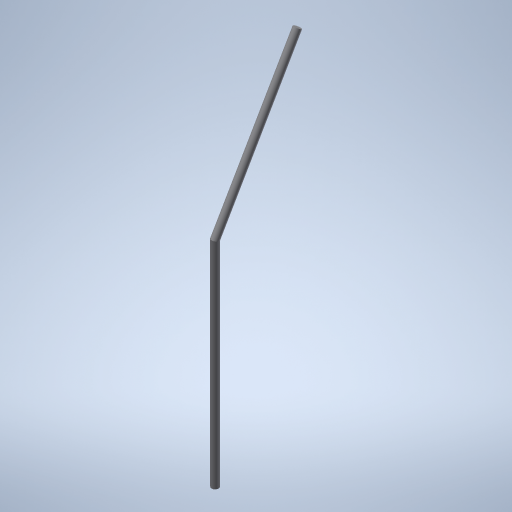
# Autodesk Inventor part: cable 30°
Saved by Autodesk Inventor 2023 (Build 270158000, 158)
## iProperties
Created: 2022-10-27
Part Number: cable 30°
Material: Generic
Document SubType Name: Modeling
Designer: Xiaba
Density: 1 g/cm^3
Appearance: Default
Author: Xiaba
Autodesk Inventor part; units mm, degrees
ref_plane "YZ Plane" through (0, 0, 0) normal (1, 0, 0) x (0, 1, 0)
ref_plane "XZ Plane" through (0, 0, 0) normal (0, 1, 0) x (-1, 0, 0)
ref_plane "XY Plane" through (0, 0, 0) normal (0, 0, 1) x (1, 0, 0)
sketch "Sketch1" plane through (0, 0, 0) normal (0, 1, 0) x (-1, 0, 0)
  circle A0 centre (0, 0) radius 0.25
  dimension "d0" = 0.5
  constraints: 1 centre point, 1 coincident
  measures "d0" diameter of A0
sketch "Sketch2" plane through (0, 0, 0) normal (1, 0, 0) x (0, 1, 0)
  line L0 (0, 0) -> (15, 0)
  line L1 (15, 0) -> (25, -5.7735)
  dimension "d1" = 15
  dimension "d2" = 150
  dimension "d3" = 10
  constraints: 4 end point, 1 horizontal
  measures "d1" distance of L0.start L0.end
  measures "d2" angle of L0 L1
  measures "d3" horizontal distance of L0.end L1.end
sweep "Sweep1" add profiles "Sketch1" path "Sketch2"
body "Solid1"
